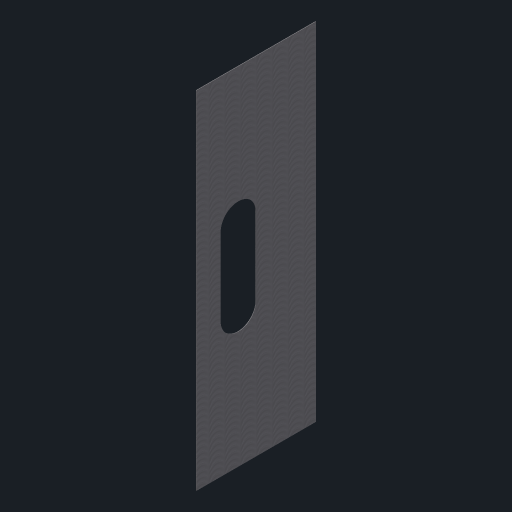
# Autodesk Inventor part: AUX_3
Saved by Autodesk Inventor 2024.3 (Build 283343000, 343)
## iProperties
Created: 2024-07-02
Part Number: AUX_3
Material: Steel, Mild, Welded
Document SubType Name: Modeling
Designer: Niler
Density: 7.85 g/cm^3
Appearance: Weld - Steel Mild
Author: Niler
Autodesk Inventor part; units mm, degrees
ref_plane "YZ Plane" through (0, 0, 0) normal (1, 0, 0) x (0, 1, 0)
ref_plane "XZ Plane" through (0, 0, 0) normal (0, 1, 0) x (-1, 0, 0)
ref_plane "XY Plane" through (0, 0, 0) normal (0, 0, 1) x (1, 0, 0)
sketch "Sketch2" plane through (0, 0, 0) normal (1, 0, 0) x (0, 1, 0)
  line L0 (107.2558, -4.179) -> (-112.7442, -4.179)
  arc A0 (-112.7442, 95.821) -> (-112.7442, -4.179) centre (-112.7442, 45.821) ccw
  line L1 (-112.7442, 95.821) -> (107.2558, 95.821)
  arc A1 (107.2558, -4.179) -> (107.2558, 95.821) centre (107.2558, 45.821) ccw
  line L2 (-494.2442, -174.3318) -> (-494.2442, 164.321)
  line L3 (488.7558, -174.3318) -> (-494.2442, -174.3318)
  line L4 (488.7558, 164.321) -> (488.7558, -174.3318)
  line L5 (-494.2442, 164.321) -> (488.7558, 164.321)
  point P0 (0, 0)
  constraints: 12 end point, 4 point on circle, 2 centre point
extrude "Extrusion1" add sketch "Sketch2" along normal blind 1.5
body "Solid1"
